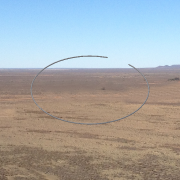
# Autodesk Inventor part: airgnd_exchange
Saved by Autodesk Inventor 2014 SP1 (Build 180222100, 222)
## iProperties
Created: 2014-03-11
Part Number: airgnd_exchange
Material: Generic
Document SubType Name: Modeling
Designer: Dave
Density: 1 g/cm^3
Appearance: Default
Author: Dave
Autodesk Inventor part; units mm, degrees
ref_plane "YZ Plane" through (0, 0, 0) normal (1, 0, 0) x (0, 1, 0)
ref_plane "XZ Plane" through (0, 0, 0) normal (0, 1, 0) x (-1, 0, 0)
ref_plane "XY Plane" through (0, 0, 0) normal (0, 0, 1) x (1, 0, 0)
sketch "Sketch1" plane through (0, 0, 0) normal (1, 0, 0) x (0, 1, 0)
  circle A0 centre (0, 0) radius 50
  circle A1 centre (0, 0) radius 45.555
  dimension "d0" = 100
  dimension "d1" = 4.445
  constraints: 2 centre point, 1 coincident
  measures "d0" diameter of A0
  measures "d1" radial gap between concentric circles of A1 A0
sketch "Sketch2" plane through (0, 0, 0) normal (0, 1, 0) x (-1, 0, 0)
  arc A0 (2329.6459, 575.8899) -> (325.3496, 10.5965) centre (0, 5000) ccw
  point P0 (0, 0)
  dimension "d2" = 10000
  dimension "d3" = 5000
  constraints: 2 point on circle, 1 centre point
  measures "d2" diameter of A0
  measures "d3" distance of point (0, 0) A0.centre
sweep "Sweep1" add profiles "Sketch1" path "Sketch2"
body "Solid1"
